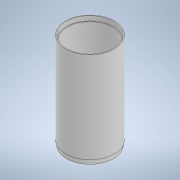
# Autodesk Inventor part: tail2
Saved by Autodesk Inventor 2020.3 (Build 243373000, 373)
## iProperties
Created: 2021-01-23
Part Number: tail2
Material: ABS Plastic
Document SubType Name: Modeling
Designer: 0x6f736f646f
Density: 1.06 g/cm^3
Appearance: Default
Mass: 73.4215 g
Surface Area: 654.885 cm^2
Volume: 69.2656 cm^3
Author: 0x6f736f646f
Autodesk Inventor part; units mm, degrees
ref_plane "YZ Plane" through (0, 0, 0) normal (1, 0, 0) x (0, 1, 0)
ref_plane "XY Plane" through (0, 0, 0) normal (0, 0, 1) x (1, 0, 0)
sketch "Sketch1" plane through (0, 0, 0) normal (0, 1, 0) x (-1, 0, 0)
  circle A0 centre (0, 0) radius 25
  circle A1 centre (0, 0) radius 25.9
  circle A2 centre (0, 0) radius 26.8
  circle A3 centre (0, 0) radius 2.5
  dimension "d0" = 50
  dimension "d1" = 51.8
  dimension "d2" = 53.6
  dimension "d33" = 5
  constraints: 4 centre point, 4 coincident
  measures "d0" diameter of A0
  measures "d1" diameter of A1
  measures "d2" diameter of A2
  measures "d33" diameter of A3
extrude "Extrusion1" add sketch "Sketch1" along normal blind 75 and the other way blind 180 contours A1
extrude "Extrusion2" add sketch "Sketch1" along normal blind 75 and the other way blind 175 contours A2
sketch "Sketch4" plane through (0, 0, 0) normal (0, 0, 1) x (1, 0, 0)
  line L0 (85, 99.9302) -> (85, 44.1135)
  line L1 (85, 44.1135) -> (25, 5)
  line L2 (25, 5) -> (25, 75)
  line L3 (25, 75) -> (85, 94.1135)
  line L4 (85, 94.1135) -> (85, 99.9302)
  line L5 (-25, 75) -> (25, 75) projected
  line L6 (-25, 75) -> (25, 75) projected
  line L7 (25.9, -180) -> (25, -180) projected
  line L8 (25, -180) -> (25, 75) projected
  line L9 (26.8, 75) -> (26.8, -175) projected
  line L10 (-25, -180) -> (-25.9, -180) projected
  line L11 (-26.8, -175) -> (-26.8, 75) projected
  line L12 (-25, 75) -> (-25, -180) projected
  line L13 (25, 75) -> (26.8, 75) projected
  line L14 (-26.8, 75) -> (-25, 75) projected
  line L15 (26.8, -175) -> (25.9, -175) projected
  line L16 (25.9, -175) -> (25.9, -180) projected
  line L17 (-25.9, -180) -> (-25.9, -175) projected
  line L18 (-25.9, -175) -> (-26.8, -175) projected
  point P0 (0, 0)
  point P1 (26.8, 96)
  point P2 (-26.8, 96)
  point P3 (26.8, 6.1734)
  point P4 (15.9, -100)
  point P5 (-15.9, -100)
  point P6 (25, 5)
  point P7 (85, 94.1135)
  dimension "d18" = 70
  dimension "d21" = 56.9
  dimension "d24" = 50
  dimension "d25" = 60
  constraints: 10 end point, 2 vertical, 1 coincident, 1 parallel, 1 point on line
  measures "d18" distance of L2.end L1.end
  measures "d21" angle of L2 L1
  measures "d24" distance of L3.end L0.end
  measures "d25" distance between parallel lines of L8 L0
extrude "Extrusion4" add sketch "Sketch4" along normal mid plane 3.6 contours L0 L1 L9 L13 L3
ref_plane "Work Plane1" through (0, -145, 0) normal (0, 1, 0) x (-1, 0, 0)
sketch "Sketch5" plane through (0, -145, 0) normal (0, 1, 0) x (-1, 0, 0)
  circle A0 centre (0, 0) radius 25
  circle A1 centre (0, 0) radius 25.9
  circle A2 centre (0, 0) radius 26.8
  circle A3 centre (0, 0) radius 2.5
  dimension "d35" = 50
  dimension "d36" = 51.8
  dimension "d37" = 53.6
  dimension "d38" = 5
  constraints: 4 centre point, 4 coincident
  measures "d35" diameter of A0
  measures "d36" diameter of A1
  measures "d37" diameter of A2
  measures "d38" diameter of A3
extrude "Extrusion5" add sketch "Sketch5" against normal blind 5 contours A0
chamfer "Chamfer1" distance 1.8 angle 45 1 edges at (55.9, 25.1435, 1.8)
chamfer "Chamfer2" distance 1.8 angle 45 1 edges at (55.9, 25.1435, -1.8)
pattern_circular "Circular Pattern3" count 3 over 360 about axis through (0, -10, 0) along (0, 1, 0) of "Extrusion4", "Chamfer2", "Chamfer1"
ref_plane "Work Plane2" through (0, -75, 0) normal (0, 1, 0) x (-1, 0, 0)
split body "Split1" result two bodies by plane through (0, -75, 0) normal (0, 1, 0) first body at (-8.8555, 25, 24.7643)
sketch "Sketch7" plane through (0, -75, 0) normal (0, -1, 0) x (1, 0, 0)
  circle A0 centre (0, 0) radius 25
  circle A1 centre (0, 0) radius 25.9
  dimension "d51" = 50
  dimension "d52" = 51.8
  constraints: 2 centre point, 2 coincident
  measures "d51" diameter of A0
  measures "d52" diameter of A1
extrude "Extrusion6" add sketch "Sketch7" along normal blind 5 bodies 2
sketch "Sketch8" plane through (0, -75, 0) normal (0, 1, 0) x (1, 0, 0)
  circle A0 centre (0, 0) radius 25
  circle A1 centre (0, 0) radius 25.9
  dimension "d55" = 50
  dimension "d56" = 51.8
  constraints: 2 centre point, 2 coincident
  measures "d55" diameter of A0
  measures "d56" diameter of A1
extrude "Extrusion7" cut sketch "Sketch8" against normal blind 5 bodies 3
body "Solid2"
body "Solid3"
